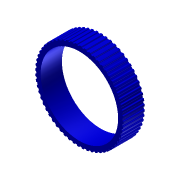
# Autodesk Inventor part: Nitrile Tread
Saved by Autodesk Inventor 2011 (Build 150239000, 239)
## iProperties
Created: 2012-06-01
Part Number: Nitrile Tread
Document SubType Name: Modeling
Designer: Nemo
Density: 1.48408 g/cm^3
Material: Rubber
Mass: 68.039 g
Surface Area: 215.07 cm^2
Volume: 45.846 cm^3
Author: Nemo
Autodesk Inventor part; units mm, degrees
ref_plane "YZ Plane" through (0, 0, 0) normal (1, 0, 0) x (0, 1, 0)
ref_plane "XZ Plane" through (0, 0, 0) normal (0, 1, 0) x (-1, 0, 0)
ref_plane "XY Plane" through (0, 0, 0) normal (0, 0, 1) x (1, 0, 0)
sketch "Sketch1" plane through (0, 0, 0) normal (0, 0, 1) x (1, 0, 0)
  circle A0 centre (0, 0) radius 46.228
  circle A1 centre (0, 0) radius 51.435
  dimension "d0" = 92.456
  dimension "d1" = 102.87
  constraints: 2 centre point, 2 coincident
  measures "d0" diameter of A0
  measures "d1" diameter of A1
extrude "Extrusion1" add sketch "Sketch1" along normal blind 25.4
sketch "Sketch2" plane through (0, 0, 25.4) normal (0, 0, 1) x (1, 0, 0)
  circle A0 centre (0, 0) radius 51.435 projected
  line L0 (0, 0) -> (0, 51.435) construction
  line L1 (0, 0) -> (0, 51.435) construction
  line L2 (0, 0) -> (0, 51.435) construction
  line L3 (2.6919, 51.3645) -> (0, 0) construction
  arc A1 (2.6919, 51.3645) -> (0, 51.435) centre (0, 0) ccw
  line L4 (0, 51.435) -> (0, 52.0661)
  line L5 (2.6919, 51.3645) -> (2.7249, 51.9948)
  arc A2 (2.1163, 52.6625) -> (0.6427, 52.7011) centre (0, 0) ccw
  arc A3 (0.6427, 52.7011) -> (0, 52.0661) centre (0.635, 52.0661) ccw
  arc A4 (2.7249, 51.9948) -> (2.1163, 52.6625) centre (2.0908, 52.028) ccw
  line L6 (0, 0) -> (5.3764, 51.1532) construction
  arc A5 (4.7522, 51.215) -> (3.3181, 51.3279) centre (0, 0) ccw
  arc A6 (2.7249, 51.9948) -> (3.3181, 51.3279) centre (3.3591, 51.9615) ccw
  line L7 (5.3764, 51.1532) -> (5.4424, 51.7809)
  arc A7 (4.7522, 51.215) -> (5.4424, 51.7809) centre (4.8109, 51.8473) ccw
  point P0 (0, 52.705)
  point P1 (2.7584, 52.6328)
  dimension "d4" = 3
  dimension "d7" = 1.27
  dimension "d8" = 0.635
  dimension "d10" = 3
  dimension "d11" = 0.635
  dimension "d12" = 0.635
  constraints: 16 end point, 16 point on circle, 8 tangent, 7 centre point, 3 coincident, 3 collinear, 3 point on line, 1 equal length, 1 equal radius, 1 vertical, 8 other
  measures "d4" angle of L2 L3
  measures "d8" radius of A3
  measures "d10" angle of L3 L6
  measures "d11" radius of A6
  measures "d12" radius of A7
extrude "Extrusion2" add sketch "Sketch2" against normal up to surface (25.4 mm away) contours A0 A7 L7 | L4 A3 A2 A4 L5 A0 | L5 A6 A0
pattern_circular "Circular Pattern1" count 60 over 360 about axis through (0, 0, 0) along (0, 0, 1) of "Extrusion2"
equation "\"d10\" = d4"
equation "\"d11\" = d8"
equation "\"d12\" = d8"
body "Solid1"
